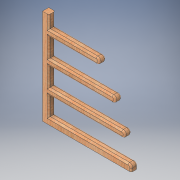
# Autodesk Inventor part: snowboard rack
Saved by Autodesk Inventor 2016 (Build 200138000, 138)
## iProperties
Created: 2017-02-05
Part Number: snowboard rack
Material: Wood (Birch)
Document SubType Name: Modeling
Designer: jwillauer
Density: 0.55 g/cm^3
Appearance: Birch - Natural Polished
Author: jwillauer
Autodesk Inventor part; units mm, degrees
ref_plane "YZ Plane" through (0, 0, 0) normal (1, 0, 0) x (0, 1, 0)
ref_plane "XZ Plane" through (0, 0, 0) normal (0, 1, 0) x (-1, 0, 0)
ref_plane "XY Plane" through (0, 0, 0) normal (0, 0, 1) x (1, 0, 0)
sketch "Sketch1" plane through (0, 0, 0) normal (0, 0, 1) x (1, 0, 0)
  line L0 (-190.2533, 169.37) -> (-164.8533, 169.37)
  line L1 (165.3467, -186.23) -> (165.3467, -211.63)
  line L2 (165.3467, -211.63) -> (-190.2533, -211.63)
  line L3 (-190.2533, -211.63) -> (-190.2533, 169.37)
  line L4 (165.3467, -186.23) -> (-164.8533, -186.23)
  line L5 (-164.8533, -186.23) -> (-164.8533, -110.03)
  line L6 (-164.8533, -110.03) -> (139.9467, -110.03)
  line L7 (139.9467, -84.63) -> (-164.8533, -84.63)
  line L8 (-164.8533, -84.63) -> (-164.8533, -8.43)
  line L9 (-164.8533, -8.43) -> (101.8467, -8.43)
  line L10 (101.8467, -8.43) -> (101.8467, 16.97)
  line L11 (101.8467, 16.97) -> (-164.8533, 16.97)
  line L12 (-164.8533, 16.97) -> (-164.8533, 93.17)
  line L13 (-164.8533, 93.17) -> (38.3467, 93.17)
  line L14 (38.3467, 93.17) -> (38.3467, 118.57)
  line L15 (38.3467, 118.57) -> (-164.8533, 118.57)
  line L16 (-164.8533, 118.57) -> (-164.8533, 169.37)
  line L17 (139.9467, -84.63) -> (139.9467, -110.03)
  point P0 (0, 0)
  dimension "d0" = 381
  dimension "d1" = 355.6
  dimension "d2" = 25.4
  dimension "d3" = 25.4
  dimension "d5" = 25.4
  dimension "d6" = 25.4
  dimension "d7" = 25.4
  dimension "d8" = 76.2
  dimension "d9" = 76.2
  dimension "d10" = 76.2
  dimension "d11" = 203.2
  dimension "d12" = 266.7
  dimension "d13" = 304.8
  constraints: 36 end point, 8 perpendicular, 5 point on line, 2 horizontal, 2 parallel, 2 vertical
  measures "d0" distance of L2.end L0.start
  measures "d1" distance of L1.end L2.end
  measures "d2" distance between parallel lines of L3 L12
  measures "d3" distance between parallel lines of L2 L4
  measures "d5" distance between parallel lines of L7 L6
  measures "d6" distance between parallel lines of L11 L9
  measures "d7" distance between parallel lines of L15 L13
  measures "d8" distance between parallel lines of L6 L4
  measures "d9" distance between parallel lines of L9 L7
  measures "d10" distance between parallel lines of L13 L11
  measures "d11" distance of L14.end L15.end
  measures "d12" distance of L10.end L11.end
  measures "d13" distance of L7.start L7.end
extrude "Extrusion1" add sketch "Sketch1" along normal blind 25.4
fillet "Fillet1" radius 12.7 5 edges at (165.3467, -186.23, 12.7) (139.9467, -84.63, 12.7) (139.9467, -110.03, 12.7) (101.8467, 16.97, 12.7) (101.8467, -8.43, 12.7)
fillet "Fillet1" radius 12.7 2 edges at (38.3467, 118.57, 12.7) (38.3467, 93.17, 12.7)
fillet "Fillet2" radius 6.35 6 edges at (34.6271, 114.8504, 25.4) (-69.6031, 93.17, 25.4) (-69.6031, 118.57, 25.4) (34.6271, 114.8504, 0) (-69.6031, 93.17, 0) (-69.6031, 118.57, 0)
fillet "Fillet3" radius 6.35 26 edges at (-164.8533, 143.97, 25.4) (-164.8533, 143.97, 0) (-164.8533, 55.07, 25.4) (-164.8533, 55.07, 0) (98.1271, 13.2504, 25.4) (-37.8531, -8.43, 25.4) (-37.8531, 16.97, 25.4) (98.1271, 13.2504, 0) (-37.8531, -8.43, 0) (-37.8531, 16.97, 0) (-164.8533, -46.53, 25.4) (-164.8533, -46.53, 0) (136.2271, -88.3496, 25.4) (-18.8031, -84.63, 25.4) (-18.8031, -110.03, 25.4) (136.2271, -88.3496, 0) (-18.8031, -110.03, 0) (-18.8031, -84.63, 0) (-164.8533, -148.13, 25.4) (-164.8533, -148.13, 0) (161.6271, -189.9496, 25.4) (165.3467, -205.2798, 25.4) (-6.1031, -186.23, 25.4) (161.6271, -189.9496, 0) (165.3467, -205.2798, 0) (-6.1031, -186.23, 0)
body "Solid1"
